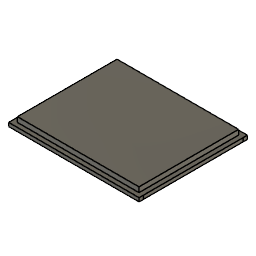
naslid (Autodesk Fusion 360 design; units mm, degrees)
Autodesk Fusion 360 part; units mm, degrees
sketch "Sketch1" plane through (0, 0, 0) normal (0, 0, 1) x (1, 0, 0)
  line L0 (0, 0) -> (71.12, 0)
  line L1 (71.12, 0) -> (71.12, -58.293)
  line L2 (71.12, -58.293) -> (0, -58.293)
  line L3 (0, -58.293) -> (0, 0)
  dimension "d1" = 71.12
  dimension "d2" = 58.293
  constraint horizontal L0
  constraint vertical L1
  constraint horizontal L2
  constraint vertical L3
  constraint coincident L0.start L3.end
  measures "d1" distance of L0.start L0.end
  measures "d2" distance of L0.start L2.end
extrude "Extrude1" add sketch "Sketch1" along normal blind 5.08 makes body 1
extrude "Extrude2" add 1 faces at (71.12, -19.431, 3.3867) along direction (1, 0, 0) blind 2.6035 separate body on bodies 1 makes body 2
extrude "Extrude3" add 1 faces at (0, -38.862, 3.3867) along direction (-1, 0, 0) blind 2.6035 separate body on bodies 1 makes body 3
extrude "Extrude4" add 1 faces at (47.4133, -58.293, 1.6933) along direction (0, -1, 0) blind 2.54 separate body on bodies 1 makes body 4
extrude "Extrude5" add 1 faces at (23.7067, 0, 1.6933) along direction (0, 1, 0) blind 2.54 separate body on bodies 1 makes body 5
extrude "Extrude6" cut 4 faces at (47.4133, -59.9863, 5.08) (-0.8678, -38.862, 5.08) (23.7067, 1.6933, 5.08) (72.8557, -19.431, 5.08) along direction (0, 0, -1) blind 1.905 on bodies 2 3 4 5 bodies 2 3 4 5
extrude "Extrude7" cut 4 faces at (72.8557, -19.431, 3.175) (23.7067, 1.6933, 3.175) (-0.8678, -38.862, 3.175) (47.4133, -59.9863, 3.175) along direction (0, 0, -1) blind 1.016 on bodies 2 3 4 5 bodies 2 3 4 5
extrude "Extrude8" add 1 faces at (71.12, -59.1397, 0.7197) along direction (1, 0, 0) blind 2.6162 on bodies 4 bodies 1 3 5 4 2
extrude "Extrude9" add 1 faces at (71.12, 0.8467, 0.7197) along direction (1, 0, 0) blind 2.6162 on bodies 5 bodies 1 3 5
extrude "Extrude10" add 1 faces at (-0.8678, 0, 0.7197) along direction (0, 1, 0) blind 2.54 on bodies 3 bodies 1 3
extrude "Extrude11" add 1 faces at (0, -59.1397, 1.4393) along direction (-1, 0, 0) blind 2.6162 on bodies 1 bodies 1
